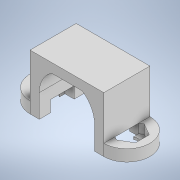
# Autodesk Inventor part: Кронштейн для двигателей серии N
Saved by Autodesk Inventor 2020 (Build 240168000, 168)
## iProperties
Created: 2019-11-25
Part Number: Кронштейн для двигателей серии N
Material: Типовые
Document SubType Name: Modeling
Designer: ivanc
Density: 1 g/cm^3
Appearance: По умолчанию
Author: ivanc
Autodesk Inventor part; units mm, degrees
ref_plane "YZ Plane" through (0, 0, 0) normal (1, 0, 0) x (0, 1, 0)
ref_plane "XZ Plane" through (0, 0, 0) normal (0, 1, 0) x (-1, 0, 0)
ref_plane "XY Plane" through (0, 0, 0) normal (0, 0, 1) x (1, 0, 0)
sketch "Эскиз1" plane through (0, 0, 0) normal (0, 0, 1) x (1, 0, 0)
  circle A0 centre (0, 0) radius 6
  line L0 (-6, 0) -> (6, 0)
  line L1 (6, 0) -> (6, 5)
  line L2 (6, 5) -> (-6, 5)
  line L3 (-6, 5) -> (-6, 0)
  line L4 (-6, 0) -> (6, 0)
  line L5 (6, 0) -> (6, -5)
  line L6 (6, -5) -> (-6, -5)
  line L7 (-6, -5) -> (-6, 0)
  line L8 (-6, -5) -> (-8, -5)
  line L9 (-8, -5) -> (-8, 5)
  line L10 (-8, 5) -> (-6, 5)
  line L11 (-6, 5) -> (-6, -5)
  line L12 (6, 5) -> (8, 5)
  line L13 (8, 5) -> (8, -5)
  line L14 (8, -5) -> (6, -5)
  line L15 (6, -5) -> (6, 5)
  line L16 (-8, 5) -> (8, 5)
  line L17 (8, 5) -> (8, 7)
  line L18 (8, 7) -> (-8, 7)
  line L19 (-8, 7) -> (-8, 5)
  line L20 (-8, -5) -> (-13, -5)
  line L21 (-13, -5) -> (-13, -2.5)
  line L22 (-13, -2.5) -> (-8, -2.5)
  line L23 (-8, -2.5) -> (-8, -5)
  line L24 (8, -5) -> (13, -5)
  line L25 (13, -5) -> (13, -2.5)
  line L26 (13, -2.5) -> (8, -2.5)
  line L27 (8, -2.5) -> (8, -5)
  point P0 (-3.3166, 5)
  point P1 (3.3166, 5)
  dimension "d0" = 12
  dimension "d1" = 5
  dimension "d2" = 5
  dimension "d3" = 2
  dimension "d4" = 2
  dimension "d5" = 2
  dimension "d8" = 5
  dimension "d9" = 5
  constraints: 56 end point, 14 parallel, 7 horizontal, 7 perpendicular, 2 point on line, 1 coincident, 3 other
  measures "d1" distance of L1.end L0.end
  measures "d2" distance of L4.end L5.end
  measures "d3" distance of L9.end L10.end
  measures "d4" distance of L13.end L14.end
  measures "d5" distance of L17.end L16.end
  measures "d8" distance of L21.end L22.end
  measures "d9" distance of L26.end L25.end
extrude "Выдавливание1" add sketch "Эскиз1" along normal blind 10 contours A0 L2 L1 | L1 L12 L13 L14 L5 | L2 A0 | A0 L2 L10 L19 L18 L17 L12 | L3 L2 A0 | L7 L8 L9 L10 L3 | L13 L26 L25 L24 | L20 L21 L22 L9
sketch "Эскиз2" plane through (-13, -2.5, 0) normal (0, 1, 0) x (1, 0, 0)
  line L0 (5, 0) -> (0, 0) projected
  line L1 (2.5, 0) -> (2.5, -10)
  line L2 (5, -10) -> (0, -10) projected
  line L3 (26, -10) -> (21, -10) projected
  line L4 (23.5, -10) -> (23.5, 0)
  line L5 (26, 0) -> (21, 0) projected
  line L6 (23.5, -5) -> (21.75, -5)
  line L7 (2.5, -5) -> (4.25, -5)
  point P0 (13, 0)
  point P1 (4.25, -5)
  dimension "d17" = 1.75
  dimension "d18" = 1.75
  constraints: 8 end point, 6 midpoint, 2 coincident, 2 horizontal
  measures "d17" distance of L6.start L6.end
  measures "d18" distance of L7.start L7.end
hole "Отверстие2" at (-8.75, -2.5, 5) at (8.75, -2.5, 5) direction (0, -1, 0) diameter 3.2 end through all
sketch "Эскиз3" plane through (8, -2.5, 0) normal (0, 1, 0) x (1, 0, 0)
  arc A0 (-16, -3.5867) -> (-16, -6.4133) centre (-16.75, -5) ccw projected
  arc A1 (0, -6.4133) -> (0, -3.5867) centre (0.75, -5) ccw projected
  line L0 (3.35, -6.5011) -> (0.75, -8.0022)
  line L1 (0.75, -8.0022) -> (-1.85, -6.5011)
  line L2 (-1.85, -6.5011) -> (-1.85, -3.4989)
  line L3 (-1.85, -3.4989) -> (0.75, -1.9978)
  line L4 (0.75, -1.9978) -> (3.35, -3.4989)
  line L5 (3.35, -3.4989) -> (3.35, -6.5011)
  line L6 (-19.35, -3.4989) -> (-16.75, -1.9978)
  line L7 (-16.75, -1.9978) -> (-14.15, -3.4989)
  line L8 (-14.15, -3.4989) -> (-14.15, -6.5011)
  line L9 (-14.15, -6.5011) -> (-16.75, -8.0022)
  line L10 (-16.75, -8.0022) -> (-19.35, -6.5011)
  line L11 (-19.35, -6.5011) -> (-19.35, -3.4989)
  line L12 (-21, 0) -> (-21, -10) projected
  line L13 (5, 0) -> (5, -10) projected
  point P0 (-8, 0)
  dimension "d26" = 5.2
  constraints: 24 end point, 3 parallel, 2 coincident, 26 other
  measures "d26" distance between parallel lines of L2 L5
extrude "Выдавливание2" cut sketch "Эскиз3" against normal blind 2
sketch "Эскиз4" plane through (6, -5, 0) normal (0, -1, 0) x (1, 0, 0)
  circle A0 centre (2.75, 5) radius 1.6 projected
  line L0 (0, 0) -> (7, 0) projected
  line L1 (7, 0) -> (7, 10) projected
  line L2 (0, 10) -> (7, 10) projected
  line L3 (0, 0) -> (0, 10) projected
  circle A1 centre (-14.75, 5) radius 1.6 projected
  line L4 (-19, 0) -> (-12, 0) projected
  line L5 (-12, 0) -> (-12, 10) projected
  line L6 (-19, 10) -> (-12, 10) projected
  line L7 (-19, 0) -> (-19, 10) projected
  circle A2 centre (-14.75, 5) radius 1.6 projected
  line L8 (-14.75, 1.9978) -> (-12.15, 3.4989) projected
  line L9 (-17.35, 3.4989) -> (-14.75, 1.9978) projected
  line L10 (-17.35, 6.5011) -> (-17.35, 3.4989) projected
  line L11 (-14.75, 8.0022) -> (-17.35, 6.5011) projected
  line L12 (-12.15, 6.5011) -> (-14.75, 8.0022) projected
  line L13 (-12.15, 3.4989) -> (-12.15, 6.5011) projected
  circle A3 centre (2.75, 5) radius 1.6 projected
  line L14 (0.15, 6.5011) -> (0.15, 3.4989) projected
  line L15 (2.75, 8.0022) -> (0.15, 6.5011) projected
  line L16 (5.35, 6.5011) -> (2.75, 8.0022) projected
  line L17 (5.35, 3.4989) -> (5.35, 6.5011) projected
  line L18 (2.75, 1.9978) -> (5.35, 3.4989) projected
  line L19 (0.15, 3.4989) -> (2.75, 1.9978) projected
  line L20 (0, 7.5692) -> (2, 7.5692)
  line L21 (2, 7.5692) -> (2, 2.4308)
  line L22 (2, 2.4308) -> (0, 2.4308)
  line L23 (0, 2.4308) -> (0, 7.5692)
  line L24 (-12, 2.4308) -> (-14, 2.4308)
  line L25 (-14, 2.4308) -> (-14, 7.5692)
  line L26 (-14, 7.5692) -> (-12, 7.5692)
  line L27 (-12, 7.5692) -> (-12, 2.4308)
  point P0 (-6, 0)
  point P1 (0, 5)
  point P2 (-12, 5)
  point P3 (0, 7.5692)
  point P4 (0, 2.4308)
  point P5 (2, 3.5867)
  point P6 (2, 6.4133)
  point P7 (-14, 6.4133)
  point P8 (-14, 3.5867)
  dimension "d29" = 2
  dimension "d30" = 2
  constraints: 16 end point, 4 midpoint, 4 parallel, 2 horizontal, 2 perpendicular, 2 point on line
  measures "d29" distance of L20.start L20.end
  measures "d30" distance of L24.start L24.end
extrude "Выдавливание3" cut sketch "Эскиз4" against normal up to surface (2.5 mm away) contours A0 L21 L19 L14 L15 | L15 L14 L19 L22 L3 L20 | A1 L25 L12 L13 L8 | L26 L5 L24 L8 L13 L12
fillet "Сопряжение1" radius 5 4 edges at (-13, -3.75, 0) (-13, -3.75, 10) (13, -3.75, 0) (13, -3.75, 10)
